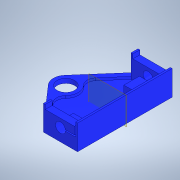
# Autodesk Inventor part: Motor Mount
Saved by Autodesk Inventor 2022 (Build 260153000, 153)
## iProperties
Created: 2022-08-10
Part Number: Motor Mount
Material: Generic
Document SubType Name: Modeling
Designer: Nick
Density: 1 g/cm^3
Appearance: Blue - Wall Paint - Glossy
Mass: 37.6373 g
Surface Area: 174.474 cm^2
Volume: 37.6373 cm^3
Author: Nick
Autodesk Inventor part; units mm, degrees
ref_plane "YZ Plane" through (0, 0, 0) normal (1, 0, 0) x (0, 1, 0)
ref_plane "XZ Plane" through (0, 0, 0) normal (0, 1, 0) x (-1, 0, 0)
ref_plane "XY Plane" through (0, 0, 0) normal (0, 0, 1) x (1, 0, 0)
sketch "Sketch14" plane through (0, 0, 0) normal (0, 0, 1) x (1, 0, 0)
  line L0 (0, 0) -> (55, 0)
  line L1 (55, 0) -> (55, 40)
  line L2 (55, 40) -> (0, 40)
  line L3 (0, 40) -> (0, 0)
  circle A0 centre (27.5, 20) radius 8
  point P0 (55, 20)
  point P1 (27.5, 40)
  dimension "d94" = 16
  dimension "d95" = 55
  dimension "d96" = 40
  constraints: 8 end point, 2 midpoint, 2 parallel, 1 centre point, 1 horizontal, 1 horizontal alignment, 1 perpendicular, 1 vertical alignment
  measures "d94" diameter of A0
  measures "d95" distance of L0.start L0.end
  measures "d96" distance of L2.end L0.start
extrude "Extrusion13" add sketch "Sketch14" along normal blind 11.26
sketch "Sketch15" plane through (0, 0, 0) normal (0, -1, 0) x (1, 0, 0)
  line L0 (0, 0) -> (55, 0) projected
  line L1 (55, 0) -> (55, 11.26) projected
  line L2 (0, 11.26) -> (55, 11.26) projected
  line L3 (0, 0) -> (0, 11.26) projected
  line L4 (55, 0) -> (55, 11.26) projected
  line L5 (55, 11.26) -> (0, 11.26)
  line L6 (0, 11.26) -> (0, 76.185)
  line L7 (0, 76.185) -> (55, 76.185)
  line L8 (55, 76.185) -> (55, 11.26)
  line L9 (0, 0) -> (0, 11.26) projected
  point P0 (0, 11.26)
  dimension "d99" = 64.925
  constraints: 8 end point, 2 parallel, 1 collinear, 1 horizontal, 1 perpendicular
  measures "d99" distance of L7.end L1.end
extrude "Extrusion14" add sketch "Sketch15" against normal blind 3 contours L6 L7 L8 L2
sketch "Sketch16" plane through (55, 0, 0) normal (1, 0, 0) x (0, 0, -1)
  line L0 (0, 0) -> (0, 40) projected
  line L1 (0, 40) -> (-11.26, 40) projected
  line L2 (-11.26, 3) -> (-11.26, 40) projected
  line L3 (-76.185, 3) -> (-11.26, 3) projected
  line L4 (-76.185, 0) -> (-76.185, 3) projected
  line L5 (0, 0) -> (-76.185, 0) projected
  line L6 (0, 40) -> (-11.26, 40) projected
  line L7 (-11.26, 3) -> (-76.185, 3) projected
  line L8 (-11.26, 3) -> (-11.26, 40) projected
  line L9 (-11.26, 40) -> (-29.0932, 40)
  line L10 (-29.0932, 40) -> (-76.185, 3)
  point P0 (0, 0)
  dimension "d106" = 29.0932
  constraints: 4 end point, 1 horizontal
  measures "d106" distance from line of L0 L9.end
extrude "Extrusion15" add sketch "Sketch16" against normal blind 3 contours L2 L3 L10 L9
ref_plane "Work Plane3" through (27.5, 0, 0) normal (1, 0, 0) x (0, 0, -1)
mirror "Mirror4" about plane through (0, 0, 76.185) normal (0, 0, 1)
sketch "Sketch18" plane through (55, 0, 0) normal (1, 0, 0) x (0, 0, -1)
  line L0 (0, 0) -> (0, 40) projected
  line L1 (0, 40) -> (-29.0932, 40) projected
  line L2 (-29.0932, 40) -> (-76.185, 3) projected
  line L3 (-123.2768, 40) -> (-76.185, 3) projected
  line L4 (-152.37, 40) -> (-123.2768, 40) projected
  line L5 (-152.37, 0) -> (-152.37, 40) projected
  line L6 (-152.37, 0) -> (0, 0) projected
  line L7 (0, 40) -> (-29.0932, 40) projected
  line L8 (-123.2768, 40) -> (-76.185, 3) projected
  line L9 (-29.0932, 40) -> (-123.2768, 40)
  point P0 (0, 0)
  constraints: 2 end point, 1 horizontal
extrude "Extrusion17" add sketch "Sketch18" against normal blind 3 contours L2 L3 L9
sketch "Sketch19" plane through (0, 0, 0) normal (0, 0, -1) x (-1, 0, 0)
  line L0 (-52, 40) -> (-3, 40)
  line L1 (-3, 40) -> (-3, 33)
  line L2 (-3, 33) -> (-52, 33)
  line L3 (-52, 33) -> (-52, 40)
  circle A0 centre (-27.5, 20) radius 8 projected
  line L4 (0, 3) -> (-52, 3) projected
  line L5 (-52, 3) -> (-52, 40) projected
  line L6 (-52, 40) -> (0, 40) projected
  line L7 (0, 40) -> (0, 3) projected
  point P0 (0, 0)
  dimension "d114" = 7
  constraints: 8 end point, 2 parallel, 1 horizontal, 1 perpendicular
  measures "d114" distance between parallel lines of L2 L0
extrude "Extrusion18" cut sketch "Sketch19" against normal through all contours L0 L1 L2 L3
sketch "Sketch20" plane through (0, 0, 0) normal (0, 0, -1) x (-1, 0, 0)
  line L0 (-27.5, 21) -> (-50, 21)
  line L1 (-50, 21) -> (-50, 33)
  line L2 (-50, 33) -> (-52, 33)
  line L3 (-52, 33) -> (-52, 19)
  line L4 (-52, 19) -> (-27.5, 19)
  line L5 (-27.5, 19) -> (-27.5, 21)
  circle A0 centre (-27.5, 20) radius 8 projected
  line L6 (-52, 33) -> (-50, 33)
  point P0 (0, 0)
  point P1 (-51, 33)
  point P2 (-35.4373, 19)
  point P3 (-35.4373, 21)
  dimension "d117" = 2
  constraints: 14 end point, 6 perpendicular, 3 midpoint, 2 coincident, 1 horizontal
  measures "d117" distance of L4.end L0.start
extrude "Extrusion19" cut sketch "Sketch20" against normal through all contours A0 L4 L3 L2 L1 L0
sketch "Sketch21" plane through (0, 3, 0) normal (0, 1, 0) x (1, 0, 0)
  line L0 (43, -11.26) -> (13.5, -11.26)
  line L1 (13.5, -11.26) -> (13.5, -36.26)
  line L2 (13.5, -36.26) -> (43, -36.26)
  line L3 (43, -36.26) -> (43, -11.26)
  line L4 (0, -141.11) -> (52, -141.11) projected
  line L5 (52, -11.26) -> (52, -141.11) projected
  line L6 (0, -11.26) -> (52, -11.26)
  line L7 (0, -11.26) -> (0, -141.11) projected
  point P0 (0, 0)
  point P1 (26, -11.26)
  dimension "d120" = 29.5
  dimension "d121" = 25
  dimension "d129" = 12.5
  constraints: 10 end point, 2 parallel, 1 horizontal, 1 midpoint, 1 perpendicular, 1 point on line
  measures "d120" distance of L1.end L2.end
  measures "d121" distance of L2.end L0.start
  measures "d129" distance from line of point (26, -11.26) L1
extrude "Extrusion20" add sketch "Sketch21" along normal blind 11.15 contours L3 L2 L1 L0
sketch "Sketch24" plane through (0, 0, 11.26) normal (0, 0, 1) x (1, 0, 0)
  line L0 (43, 14.15) -> (43, 3) projected
  line L1 (43, 3) -> (52, 3) projected
  line L2 (52, 3) -> (52, 19) projected
  line L3 (52, 19) -> (35.4373, 19) projected
  arc A0 (32.9569, 14.15) -> (35.4373, 19) centre (27.5, 20) ccw projected
  line L4 (32.9569, 14.15) -> (43, 14.15) projected
  line L5 (43, 14.15) -> (43, 19)
  line L6 (52, 19) -> (35.4373, 19) projected
  point P0 (0, 0)
  constraints: 2 end point, 1 perpendicular, 1 point on line
extrude "Extrusion23" add sketch "Sketch24" along normal up to surface (25 mm away) contours L4 A0 L3 L5
ref_plane "Work Plane4" through (0, 0, 76.185) normal (0, 0, -1) x (-1, 0, 0)
sketch "Sketch25" plane through (0, 3, 0) normal (0, 1, 0) x (1, 0, 0)
  line L0 (40, -141.11) -> (12, -141.11)
  line L1 (12, -141.11) -> (12, -116.11)
  line L2 (12, -116.11) -> (40, -116.11)
  line L3 (40, -116.11) -> (40, -141.11)
  line L4 (0, -141.11) -> (52, -141.11) projected
  point P0 (0, 0)
  point P1 (26, -141.11)
  dimension "d132" = 25
  dimension "d133" = 28
  constraints: 8 end point, 2 midpoint, 2 parallel, 1 horizontal, 1 perpendicular
  measures "d132" distance of L2.end L0.start
  measures "d133" distance of L1.end L2.end
extrude "Extrusion24" add sketch "Sketch25" along normal blind 11.15
sketch "Sketch26" plane through (0, 0, 0) normal (0, -1, 0) x (1, 0, 0)
  line L0 (0, 0) -> (55, 0) projected
  line L1 (0, 0) -> (-55.0618, 63.0266)
  line L2 (0, 152.37) -> (-55.0618, 89.3434)
  arc A0 (-55.0618, 89.3434) -> (-55.0618, 63.0266) centre (-40, 76.185) ccw
  line L3 (0, 0) -> (0, 152.37) projected
  line L4 (0, 0) -> (0, 152.37)
  circle A1 centre (-40, 76.185) radius 14
  point P0 (0, 44.2511)
  point P1 (0, 44.2511)
  dimension "d137" = 20
  dimension "d138" = 40
  dimension "d146" = 28
  constraints: 6 end point, 2 centre point, 2 point on circle, 2 tangent, 1 coincident, 1 equal length, 1 vertical
  measures "d137" radius of A0
  measures "d138" distance from line of L3 A0.centre
  measures "d146" diameter of A1
extrude "Extrusion25" add sketch "Sketch26" against normal blind 3
sketch "Sketch27" plane through (0, 3, 0) normal (0, 1, 0) x (1, 0, 0)
  arc A0 (-55.0618, -63.0266) -> (-55.0618, -89.3434) centre (-40, -76.185) ccw projected
  circle A1 centre (-40, -76.185) radius 14
  circle A2 centre (-40, -76.185) radius 20
  line L0 (0, 0) -> (-55.0618, -63.0266) projected
  line L1 (-55.0618, -89.3434) -> (0, -152.37) projected
  line L2 (3, -141.11) -> (0, -141.11) projected
  line L3 (-26.5102, -110.765) -> (0, -141.11)
  line L4 (0, -11.26) -> (-26.5102, -41.605)
  arc A3 (-26.5102, -41.605) -> (-25.8365, -62.0643) centre (-15.2138, -51.4737) ccw
  arc A4 (-25.8365, -90.3057) -> (-26.5102, -110.765) centre (-15.2138, -100.8963) ccw
  line L5 (-55.0618, -63.0266) -> (0, 0) projected
  line L6 (0, 0) -> (0, -11.26)
  line L7 (0, -141.11) -> (12, -141.11) projected
  line L8 (0, -152.37) -> (0, -141.11) projected
  line L9 (0, -141.11) -> (0, -152.37)
  point P0 (-32.2708, -36.9389)
  point P1 (-29.1283, -59.3979)
  point P2 (-29.1283, -92.9721)
  point P3 (-32.2708, -115.4311)
  point P4 (-55.0618, -63.0266)
  dimension "d141" = 28
  dimension "d145" = 15
  constraints: 9 point on circle, 8 end point, 4 centre point, 4 tangent, 2 coincident, 2 parallel, 2 point on line, 1 collinear, 1 equal radius, 1 vertical
  measures "d141" diameter of A1
  measures "d145" radius of A3
extrude "Extrusion26" add sketch "Sketch27" along normal blind 4
sketch "Sketch28" plane through (52, 19, 141.11) normal (0, 0, -1) x (-1, 0, 0)
  line L0 (12, -16) -> (12, -4.85) projected
  line L1 (12, -4.85) -> (19.0431, -4.85) projected
  arc A0 (16.5627, 0) -> (19.0431, -4.85) centre (24.5, 1) ccw projected
  line L2 (16.5627, 0) -> (0, 0) projected
  line L3 (0, -16) -> (0, 0) projected
  line L4 (12, -16) -> (0, -16) projected
  line L5 (12, -16) -> (12, -4.85) projected
  line L6 (12, -4.85) -> (12, 0)
  line L7 (16.5627, 0) -> (0, 0) projected
  point P0 (52, -19)
  point P1 (12, 0)
  constraints: 2 end point, 1 perpendicular, 1 point on line
extrude "Extrusion27" add sketch "Sketch28" along normal up to surface (25 mm away) contours L6 L2 A0 L1
sketch "Sketch29" plane through (0, 3, 0) normal (0, 1, 0) x (1, 0, 0)
  circle A0 centre (-0.5, -30.26) radius 14
  line L0 (13.5, -11.26) -> (13.5, -36.26) projected
  line L1 (50, -11.26) -> (3, -11.26) projected
  circle A1 centre (-0.5, -30.26) radius 10
  point P0 (0, 0)
  dimension "d149" = 28
  dimension "d150" = 19
  dimension "d151" = 20
  constraints: 2 centre point, 1 coincident, 1 tangent
  measures "d149" diameter of A0
  measures "d150" distance from line of A0.centre L1
  measures "d151" diameter of A1
extrude "Extrusion28" cut sketch "Sketch29" against normal blind 10 contours A1
body "Solid3"
